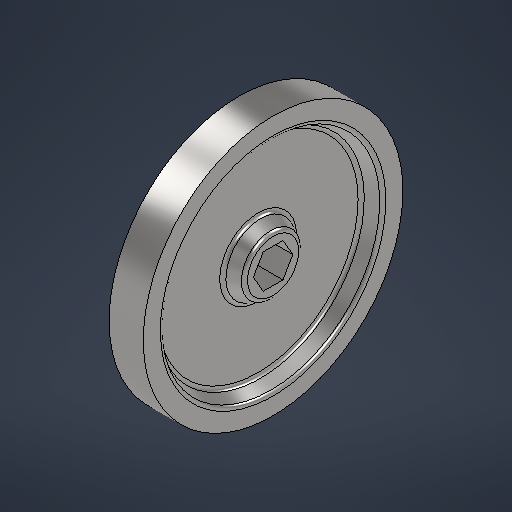
# Autodesk Inventor part: Shooter,FlyWheel
Saved by Autodesk Inventor 2026.1 (Build 301233020, 233B)
## iProperties
Created: 2026-01-18
Part Number: Shooter,FlyWheel
Material: Steel, Alloy
Document SubType Name: Modeling
Designer: Owen L
Mass: 321.181 g
Surface Area: 207.112 cm^2
Volume: 41.5499 cm^3
Density: 7.73 g/cm^3
Appearance: Semi-Polished
Author: Owen L
Autodesk Inventor part; units mm, degrees
ref_plane "YZ Plane" through (0, 0, 0) normal (1, 0, 0) x (0, 1, 0)
ref_plane "XZ Plane" through (0, 0, 0) normal (0, 1, 0) x (-1, 0, 0)
ref_plane "XY Plane" through (0, 0, 0) normal (0, 0, 1) x (1, 0, 0)
sketch "Sketch3" plane through (0, 0, 0) normal (0, 0, 1) x (1, 0, 0)
  line L0 (-7.8604, 0) -> (1.3101, 0) projected
  line L1 (0, -9.652) -> (0, 57.912) projected
  line L2 (-6.35, 0) -> (-6.35, 9.525)
  line L3 (-5.479, 10.9416) -> (-1.6647, 12.8709)
  line L4 (-0.7938, 14.2875) -> (-0.7938, 37.1475)
  line L5 (-6.35, 41.91) -> (-6.35, 48.26)
  line L6 (-6.35, 48.26) -> (0, 48.26)
  arc A0 (-0.7938, 37.1475) -> (-1.6647, 38.5641) centre (-2.3813, 37.1475) ccw
  arc A1 (-1.6647, 12.8709) -> (-0.7938, 14.2875) centre (-2.3813, 14.2875) ccw
  arc A2 (-5.479, 10.9416) -> (-6.35, 9.525) centre (-4.7625, 9.525) ccw
  arc A3 (-6.35, 41.91) -> (-5.479, 40.4934) centre (-4.7625, 41.91) ccw
  line L7 (-5.479, 40.4934) -> (-1.6647, 38.5641)
  point P0 (0, 0)
  point P1 (-6.35, 37.836)
  dimension "d14" = 6.35
  dimension "d15" = 1.5875
  dimension "d16" = 12.7
  dimension "d18" = 19.05
  dimension "d19" = 96.52
  dimension "d21" = 1.5875
  dimension "d22" = 1.5875
  dimension "d23" = 28.575
  dimension "d24" = 6.35
  constraints: 12 end point, 8 point on circle, 8 tangent, 4 centre point, 3 point on line, 2 equal radius, 2 perpendicular, 1 equal length, 1 parallel, 1 vertical
  measures "d14" distance of L5.end L6.end
  measures "d15" diameter of L4 L1
  measures "d16" diameter of L2 L1
  measures "d18" diameter of L2.end L0
  measures "d19" diameter of L6 L0
  measures "d21" radius of A3
  measures "d22" radius of A1
  measures "d23" diameter of L4.start L0
  measures "d24" distance from line of L5.start L6
revolve "Revolution1" add sketch "Sketch3" angle 360 about axis through (-10, 0, 0) along (1, 0, 0)
mirror "Mirror1" about plane through (0, 0, 0) normal (1, 0, 0) of "Revolution1"
sketch "Sketch4" plane through (-6.35, 0, 0) normal (-1, 0, 0) x (0, 0, 1)
  line L0 (3.6662, -6.35) -> (-3.6662, -6.35)
  line L1 (-3.6662, -6.35) -> (-7.3323, 0)
  line L2 (-7.3323, 0) -> (-3.6662, 6.35)
  line L3 (-3.6662, 6.35) -> (3.6662, 6.35)
  line L4 (3.6662, 6.35) -> (7.3323, 0)
  line L5 (7.3323, 0) -> (3.6662, -6.35)
  point P0 (0, 0)
  point P1 (0, 0)
  dimension "d26" = 12.7
  constraints: 12 end point, 1 coincident, 1 horizontal, 13 other
  measures "d26" distance between parallel lines of L3 L0
extrude "Extrusion2" cut sketch "Sketch4" against normal through all
body "Solid2"
